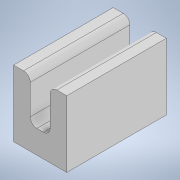
# Autodesk Inventor part: koppelstuk
Saved by Autodesk Inventor 2021 (Build 250183000, 183)
## iProperties
Created: 2023-10-11
Part Number: koppelstuk
Material: Generic
Document SubType Name: Modeling
Designer: Elias
Density: 1 g/cm^3
Appearance: Default
Author: Elias
Autodesk Inventor part; units mm, degrees
ref_plane "YZ Plane" through (0, 0, 0) normal (1, 0, 0) x (0, 1, 0)
ref_plane "XZ Plane" through (0, 0, 0) normal (0, 1, 0) x (-1, 0, 0)
ref_plane "XY Plane" through (0, 0, 0) normal (0, 0, 1) x (1, 0, 0)
sketch "Sketch1" plane through (0, 0, 0) normal (0, 0, 1) x (1, 0, 0)
  line L0 (0, 0) -> (8, 0)
  line L1 (8, 0) -> (8, 10)
  line L2 (8, 10) -> (0, 10)
  line L3 (0, 10) -> (0, 0)
  dimension "d0" = 8
  dimension "d1" = 10
  constraints: 8 end point, 2 parallel, 1 horizontal, 1 perpendicular
  measures "d0" distance of L1.end L2.end
  measures "d1" distance of L0.end L1.end
extrude "Extrusion1" add sketch "Sketch1" along normal blind 15
sketch "Sketch2" plane through (0, 0, 15) normal (0, 0, 1) x (1, 0, 0)
  line L0 (8, 10) -> (0, 10) projected
  line L1 (2.5, 10) -> (5.5, 10)
  line L2 (5.5, 10) -> (5.5, 3.5)
  line L3 (5.5, 3.5) -> (2.5, 3.5)
  line L4 (2.5, 3.5) -> (2.5, 10)
  line L5 (0, 10) -> (0, 0) projected
  line L6 (8, 0) -> (8, 10) projected
  line L7 (0, 0) -> (8, 0) projected
  dimension "d4" = 2.5
  dimension "d5" = 2.5
  dimension "d6" = 3.5
  constraints: 8 end point, 2 parallel, 1 horizontal, 1 perpendicular, 1 point on line
  measures "d4" distance between parallel lines of L5 L4
  measures "d5" distance between parallel lines of L6 L2
  measures "d6" distance between parallel lines of L7 L3
extrude "Extrusion2" cut sketch "Sketch2" against normal blind 15 contours L2 L3 L4 L0
fillet "Fillet2" radius 1 4 edges at (2.5, 10, 7.5) (5.5, 10, 7.5) (2.5, 3.5, 7.5) (5.5, 3.5, 7.5)
body "Solid1"
